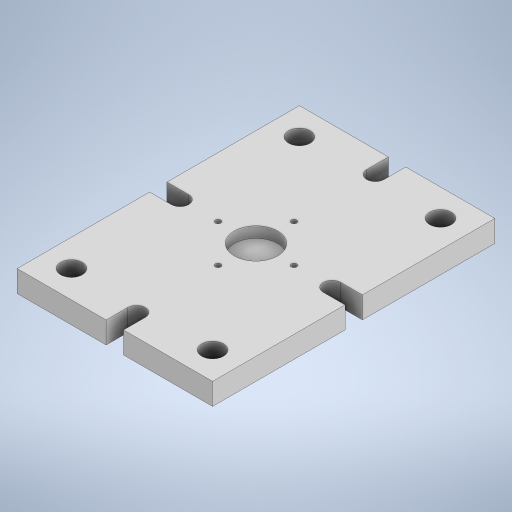
# Autodesk Inventor part: Base inferior da ferramenta
Saved by Autodesk Inventor 2023 (Build 270158000, 158)
## iProperties
Created: 2022-04-24
Part Number: Base inferior da ferramenta
Material: Generic
Document SubType Name: Modeling
Designer: coqui
Density: 1 g/cm^3
Appearance: Default
Author: coqui
Autodesk Inventor part; units mm, degrees
ref_plane "YZ Plane" through (0, 0, 0) normal (1, 0, 0) x (0, 1, 0)
ref_plane "XZ Plane" through (0, 0, 0) normal (0, 1, 0) x (-1, 0, 0)
ref_plane "XY Plane" through (0, 0, 0) normal (0, 0, 1) x (1, 0, 0)
sketch "Sketch2" plane through (0, 0, 0) normal (0, 1, 0) x (-1, 0, 0)
  line L0 (90, 130) -> (-90, -130) construction
  line L1 (-90, 130) -> (90, -130) construction
  circle A0 centre (65, 105) radius 10
  circle A1 centre (-65, 105) radius 10
  circle A2 centre (-65, -105) radius 10
  circle A3 centre (65, -105) radius 10
  line L2 (0, 65.8121) -> (0, -50.2865) construction
  line L3 (90, 0) -> (70, 0) construction
  line L4 (90, -8) -> (70, -8)
  line L5 (70, 8) -> (90, 8)
  arc A4 (70, 8) -> (70, -8) centre (70, 0) ccw
  line L6 (-90, -8) -> (-70, -8)
  line L7 (-70, 8) -> (-90, 8)
  arc A5 (-70, -8) -> (-70, 8) centre (-70, 0) ccw
  line L8 (90, -130) -> (90, -8)
  line L9 (90, 8) -> (90, 130)
  line L10 (-90, 130) -> (-90, 8)
  line L11 (-90, -8) -> (-90, -130)
  line L12 (0, -110) -> (0, -154.4719) construction
  line L13 (-8, -110) -> (-8, -130)
  line L14 (8, -130) -> (8, -110)
  arc A6 (8, -110) -> (-8, -110) centre (0, -110) ccw
  line L15 (25.1981, 0) -> (-33.3058, 0) construction
  line L16 (-8, 110) -> (-8, 130)
  line L17 (8, 130) -> (8, 110)
  arc A7 (-8, 110) -> (8, 110) centre (0, 110) ccw
  line L18 (90, 130) -> (8, 130)
  line L19 (-8, 130) -> (-90, 130)
  line L20 (-90, -130) -> (-8, -130)
  line L21 (8, -130) -> (90, -130)
  point P0 (0, 0)
  point P1 (80, 0)
  point P2 (0, -132.2359)
  point P3 (8, 154.4719)
  dimension "d2" = 180
  dimension "d3" = 260
  dimension "d4" = 20
  dimension "d6" = 65
  dimension "d7" = 65
  dimension "d9" = 65
  dimension "d12" = 65
  dimension "d16" = 8
  dimension "d18" = 8
  constraints: 48 end point, 10 parallel, 8 centre point, 8 point on circle, 8 symmetric about line, 4 horizontal, 4 midpoint, 4 perpendicular, 4 tangent, 3 equal radius, 2 horizontal alignment, 2 vertical, 2 vertical alignment, 2 other
  measures "d2" distance of L1.end L0.end
  measures "d3" distance of L1.start L0.end
  measures "d4" diameter of A0
  measures "d6" horizontal distance of A0.centre point (0, 0)
  measures "d7" horizontal distance of point (0, 0) A3.centre
  measures "d9" horizontal distance of A1.centre point (0, 0)
  measures "d12" horizontal distance of A2.centre point (0, 0)
  measures "d16" radius of A4
  measures "d18" radius of A6
extrude "Extrusion2" add sketch "Sketch2" along normal blind 20
sketch "Sketch3" plane through (0, 20, 0) normal (0, 1, 0) x (1, 0, 0)
  circle A0 centre (0, 35) radius 2.5
  circle A1 centre (-35, 0) radius 2.5
  circle A2 centre (0, -35) radius 2.5
  circle A3 centre (35, 0) radius 2.5
  point P0 (0, 0)
  dimension "d22" = 5
  dimension "d23" = 35
  dimension "d26" = 360
  constraints: 4 centre point, 9 other
  measures "d22" diameter of A0
  measures "d23" distance of point (0, 0) A0.centre
extrude "Extrusion3" cut sketch "Sketch3" against normal blind 12
sketch "Sketch4" plane through (0, 20, 0) normal (0, 1, 0) x (1, 0, 0)
  circle A0 centre (0, 0) radius 20
  dimension "d30" = 40
  constraints: 1 centre point, 1 coincident
  measures "d30" diameter of A0
extrude "Extrusion4" cut sketch "Sketch4" against normal blind 10
body "Solid2"
